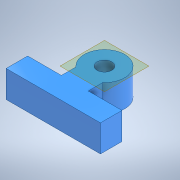
# Autodesk Inventor part: 4mm_Roller_Spacer
Saved by Autodesk Inventor 2021 (Build 250183000, 183)
## iProperties
Created: 2021-03-29
Part Number: 4mm_Roller_Spacer
Material: PET Plastic
Document SubType Name: Modeling
Designer: Jorian Brusind
Density: 1.541 g/cm^3
Appearance: Cyan
Author: Jorian Brusind
Autodesk Inventor part; units mm, degrees
ref_plane "YZ Plane" through (0, 0, 0) normal (1, 0, 0) x (0, 1, 0)
ref_plane "XZ Plane" through (0, 0, 0) normal (0, 1, 0) x (-1, 0, 0)
ref_plane "XY Plane" through (0, 0, 0) normal (0, 0, 1) x (1, 0, 0)
sketch "Sketch4" plane through (0, 0, 0) normal (0, 1, 0) x (-1, 0, 0)
  circle A0 centre (0, 0) radius 7.5
  circle A1 centre (0, 0) radius 2.75
  dimension "d19" = 15
  dimension "d20" = 5.5
  constraints: 2 centre point, 2 coincident
  measures "d19" diameter of A0
  measures "d20" diameter of A1
extrude "Extrusion4" add sketch "Sketch4" along normal blind 10
ref_plane "Work Plane1" through (0, 10, 0) normal (0, -1, 0) x (1, 0, 0)
sketch "Sketch7" plane through (0, 10, 0) normal (0, -1, 0) x (1, 0, 0)
  line L0 (0, 0) -> (0, 15)
  line L1 (17.5, 19) -> (-17.5, 19)
  line L2 (-17.5, 19) -> (-17.5, 11)
  line L3 (-17.5, 11) -> (17.5, 11)
  line L4 (17.5, 11) -> (17.5, 19)
  line L5 (17.5, 19) -> (-17.5, 11) construction
  line L6 (-17.5, 19) -> (17.5, 11) construction
  line L7 (5, 24.41) -> (-5, 24.41)
  line L8 (-5, 24.41) -> (-5, 5.59)
  line L9 (-5, 5.59) -> (5, 5.59)
  line L10 (5, 5.59) -> (5, 24.41)
  line L11 (5, 24.41) -> (-5, 5.59) construction
  line L12 (-5, 24.41) -> (5, 5.59) construction
  point P0 (-5, 11)
  point P1 (5, 11)
  dimension "d35" = 15
  dimension "d36" = 35
  dimension "d37" = 8
  dimension "d38" = 10
  dimension "d39" = 18.82
  constraints: 26 end point, 4 midpoint, 4 parallel, 2 horizontal, 2 perpendicular, 1 vertical
  measures "d35" distance of L0.start L0.end
  measures "d36" distance of L3.end L2.end
  measures "d37" distance of L2.end L1.end
  measures "d38" distance of L9.end L8.end
  measures "d39" distance of L8.end L7.end
extrude "Extrusion6" add sketch "Sketch7" along normal up to surface (10 mm away) contours L9 L8 L3 L0 | L0 L3 L10 L9 | L3 L8 L1 L10 | L3 L2 L1 L8 | L10 L1 L4 L3
body "Solid2"
